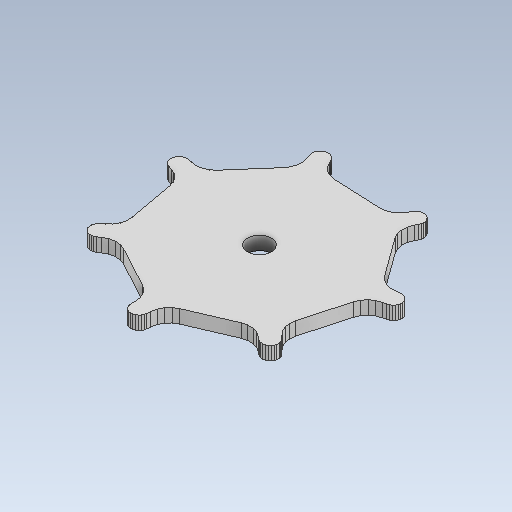
# Autodesk Inventor part: sprocket7
Saved by Autodesk Inventor 2020 (Build 240168000, 168)
## iProperties
Created: 2019-07-16
Part Number: sprocket7
Material: Generic
Document SubType Name: Modeling
Designer: erwin
Density: 1 g/cm^3
Appearance: Default
Mass: 305.43 g
Surface Area: 609.721 cm^2
Volume: 305.43 cm^3
Author: erwin
Autodesk Inventor part; units mm, degrees
ref_plane "YZ Plane" through (0, 0, 0) normal (1, 0, 0) x (0, 1, 0)
ref_plane "XZ Plane" through (0, 0, 0) normal (0, 1, 0) x (-1, 0, 0)
ref_plane "XY Plane" through (0, 0, 0) normal (0, 0, 1) x (1, 0, 0)
sketch "Sketch2" plane through (0, 0, 0) normal (0, 1, 0) x (-1, 0, 0)
  line L0 (77.8598, 129.5505) -> (181.2412, 129.5505)
  line L1 (129.5505, 77.8598) -> (129.5505, 181.2412)
  line L2 (208.1814, 165.1629) -> (207.9893, 170.0518)
  line L3 (207.9893, 170.0518) -> (209.1581, 174.8028)
  line L4 (209.1581, 174.8028) -> (211.5965, 179.0445)
  line L5 (211.5965, 179.0445) -> (215.1139, 182.4454)
  line L6 (215.1139, 182.4454) -> (217.4859, 184.4007)
  line L7 (217.4859, 184.4007) -> (218.8706, 185.7147)
  line L8 (218.8706, 185.7147) -> (219.868, 187.3423)
  line L9 (219.868, 187.3423) -> (220.4102, 189.1727)
  line L10 (220.4102, 189.1727) -> (220.4602, 191.0809)
  line L11 (220.4602, 191.0809) -> (220.0145, 192.9371)
  line L12 (220.0145, 192.9371) -> (219.1037, 194.6147)
  line L13 (219.1037, 194.6147) -> (217.7897, 195.9994)
  line L14 (217.7897, 195.9994) -> (216.162, 196.9968)
  line L15 (216.162, 196.9968) -> (214.3317, 197.5389)
  line L16 (214.3317, 197.5389) -> (212.4235, 197.5889)
  line L17 (212.4235, 197.5889) -> (210.5673, 197.1433)
  line L18 (210.5673, 197.1433) -> (208.8897, 196.2324)
  line L19 (208.8897, 196.2324) -> (206.2971, 194.5807)
  line L20 (206.2971, 194.5807) -> (201.9757, 192.2864)
  line L21 (201.9757, 192.2864) -> (197.1881, 191.2781)
  line L22 (197.1881, 191.2781) -> (192.3084, 191.6346)
  line L23 (192.3084, 191.6346) -> (187.7182, 193.3281)
  line L24 (187.7182, 193.3281) -> (150.7331, 213.2305)
  line L25 (150.7331, 213.2305) -> (146.7911, 216.1285)
  line L26 (146.7911, 216.1285) -> (143.8054, 220.0046)
  line L27 (143.8054, 220.0046) -> (142.0094, 224.5557)
  line L28 (142.0094, 224.5557) -> (141.5435, 229.4261)
  line L29 (141.5435, 229.4261) -> (141.4937, 232.4997)
  line L30 (141.4937, 232.4997) -> (141.3297, 234.4016)
  line L31 (141.3297, 234.4016) -> (140.6791, 236.1962)
  line L32 (140.6791, 236.1962) -> (139.5861, 237.7613)
  line L33 (139.5861, 237.7613) -> (138.1253, 238.9901)
  line L34 (138.1253, 238.9901) -> (136.3963, 239.799)
  line L35 (136.3963, 239.799) -> (134.5168, 240.1329)
  line L36 (134.5168, 240.1329) -> (132.6149, 239.9689)
  line L37 (132.6149, 239.9689) -> (130.8203, 239.3182)
  line L38 (130.8203, 239.3182) -> (129.2552, 238.2252)
  line L39 (129.2552, 238.2252) -> (128.0264, 236.7645)
  line L40 (128.0264, 236.7645) -> (127.2175, 235.0354)
  line L41 (127.2175, 235.0354) -> (126.8836, 233.1559)
  line L42 (126.8836, 233.1559) -> (126.5586, 230.0991)
  line L43 (126.5586, 230.0991) -> (125.658, 225.29)
  line L44 (125.658, 225.29) -> (123.4612, 220.9182)
  line L45 (123.4612, 220.9182) -> (120.1401, 217.3254)
  line L46 (120.1401, 217.3254) -> (115.9541, 214.7925)
  line L47 (115.9541, 214.7925) -> (77.334, 198.2854)
  line L48 (77.334, 198.2854) -> (72.6104, 197.0103)
  line L49 (72.6104, 197.0103) -> (67.7184, 197.0926)
  line L50 (67.7184, 197.0926) -> (63.0404, 198.526)
  line L51 (63.0404, 198.526) -> (58.9421, 201.1984)
  line L52 (58.9421, 201.1984) -> (56.508, 203.0759)
  line L53 (56.508, 203.0759) -> (54.9188, 204.1335)
  line L54 (54.9188, 204.1335) -> (53.1101, 204.7437)
  line L55 (53.1101, 204.7437) -> (51.205, 204.865)
  line L56 (51.205, 204.865) -> (49.3334, 204.4891)
  line L57 (49.3334, 204.4891) -> (47.623, 203.6416)
  line L58 (47.623, 203.6416) -> (46.1901, 202.3802)
  line L59 (46.1901, 202.3802) -> (45.1326, 200.7911)
  line L60 (45.1326, 200.7911) -> (44.5223, 198.9823)
  line L61 (44.5223, 198.9823) -> (44.401, 197.0772)
  line L62 (44.401, 197.0772) -> (44.777, 195.2057)
  line L63 (44.777, 195.2057) -> (45.6245, 193.4952)
  line L64 (45.6245, 193.4952) -> (46.8858, 192.0624)
  line L65 (46.8858, 192.0624) -> (49.073, 189.9023)
  line L66 (49.073, 189.9023) -> (52.2714, 186.1998)
  line L67 (52.2714, 186.1998) -> (54.3197, 181.7566)
  line L68 (54.3197, 181.7566) -> (55.058, 176.9199)
  line L69 (55.058, 176.9199) -> (54.4284, 172.0679)
  line L70 (54.4284, 172.0679) -> (43.2549, 131.5815)
  line L71 (43.2549, 131.5815) -> (41.3067, 127.0934)
  line L72 (41.3067, 127.0934) -> (38.1923, 123.3201)
  line L73 (38.1923, 123.3201) -> (34.1549, 120.5564)
  line L74 (34.1549, 120.5564) -> (29.5103, 119.0184)
  line L75 (29.5103, 119.0184) -> (26.5248, 118.2859)
  line L76 (26.5248, 118.2859) -> (24.7071, 117.7028)
  line L77 (24.7071, 117.7028) -> (23.1023, 116.6692)
  line L78 (23.1023, 116.6692) -> (21.8196, 115.2553)
  line L79 (21.8196, 115.2553) -> (20.9467, 113.5577)
  line L80 (20.9467, 113.5577) -> (20.5428, 111.692)
  line L81 (20.5428, 111.692) -> (20.6356, 109.7853)
  line L82 (20.6356, 109.7853) -> (21.2187, 107.9677)
  line L83 (21.2187, 107.9677) -> (22.2523, 106.3628)
  line L84 (22.2523, 106.3628) -> (23.6661, 105.0802)
  line L85 (23.6661, 105.0802) -> (25.3638, 104.2072)
  line L86 (25.3638, 104.2072) -> (27.2295, 103.8034)
  line L87 (27.2295, 103.8034) -> (29.1361, 103.8961)
  line L88 (29.1361, 103.8961) -> (32.1886, 104.2594)
  line L89 (32.1886, 104.2594) -> (37.0775, 104.4515)
  line L90 (37.0775, 104.4515) -> (41.8285, 103.2827)
  line L91 (41.8285, 103.2827) -> (46.0703, 100.8443)
  line L92 (46.0703, 100.8443) -> (49.4712, 97.3269)
  line L93 (49.4712, 97.3269) -> (74.1582, 63.3482)
  line L94 (74.1582, 63.3482) -> (76.4524, 59.0268)
  line L95 (76.4524, 59.0268) -> (77.4607, 54.2392)
  line L96 (77.4607, 54.2392) -> (77.1042, 49.3595)
  line L97 (77.1042, 49.3595) -> (75.4108, 44.7692)
  line L98 (75.4108, 44.7692) -> (74.122, 41.9784)
  line L99 (74.122, 41.9784) -> (73.4446, 40.1937)
  line L100 (73.4446, 40.1937) -> (73.2521, 38.2945)
  line L101 (73.2521, 38.2945) -> (73.5578, 36.4102)
  line L102 (73.5578, 36.4102) -> (74.3407, 34.6693)
  line L103 (74.3407, 34.6693) -> (75.5476, 33.1902)
  line L104 (75.5476, 33.1902) -> (77.0961, 32.074)
  line L105 (77.0961, 32.074) -> (78.8808, 31.3966)
  line L106 (78.8808, 31.3966) -> (80.78, 31.2041)
  line L107 (80.78, 31.2041) -> (82.6643, 31.5098)
  line L108 (82.6643, 31.5098) -> (84.4053, 32.2927)
  line L109 (84.4053, 32.2927) -> (85.8843, 33.4996)
  line L110 (85.8843, 33.4996) -> (87.0006, 35.0481)
  line L111 (87.0006, 35.0481) -> (88.6197, 37.6612)
  line L112 (88.6197, 37.6612) -> (91.5177, 41.6033)
  line L113 (91.5177, 41.6033) -> (95.3937, 44.589)
  line L114 (95.3937, 44.589) -> (99.9449, 46.385)
  line L115 (99.9449, 46.385) -> (104.8153, 46.8509)
  line L116 (104.8153, 46.8509) -> (146.773, 44.9666)
  line L117 (146.773, 44.9666) -> (151.582, 44.066)
  line L118 (151.582, 44.066) -> (155.9538, 41.8692)
  line L119 (155.9538, 41.8692) -> (159.5466, 38.5481)
  line L120 (159.5466, 38.5481) -> (162.0796, 34.3621)
  line L121 (162.0796, 34.3621) -> (163.458, 31.6144)
  line L122 (163.458, 31.6144) -> (164.431, 29.9721)
  line L123 (164.431, 29.9721) -> (165.7958, 28.6375)
  line L124 (165.7958, 28.6375) -> (167.4596, 27.7016)
  line L125 (167.4596, 27.7016) -> (169.3089, 27.2283)
  line L126 (169.3089, 27.2283) -> (171.2177, 27.2497)
  line L127 (171.2177, 27.2497) -> (173.0559, 27.7644)
  line L128 (173.0559, 27.7644) -> (174.6983, 28.7374)
  line L129 (174.6983, 28.7374) -> (176.0329, 30.1023)
  line L130 (176.0329, 30.1023) -> (176.9687, 31.766)
  line L131 (176.9687, 31.766) -> (177.4421, 33.6153)
  line L132 (177.4421, 33.6153) -> (177.4207, 35.5241)
  line L133 (177.4207, 35.5241) -> (176.9059, 37.3624)
  line L134 (176.9059, 37.3624) -> (175.8725, 40.2575)
  line L135 (175.8725, 40.2575) -> (174.5974, 44.9811)
  line L136 (174.5974, 44.9811) -> (174.6797, 49.873)
  line L137 (174.6797, 49.873) -> (176.1131, 54.551)
  line L138 (176.1131, 54.551) -> (178.7855, 58.6494)
  line L139 (178.7855, 58.6494) -> (206.4189, 90.2784)
  line L140 (206.4189, 90.2784) -> (210.1214, 93.4767)
  line L141 (210.1214, 93.4767) -> (214.5647, 95.5251)
  line L142 (214.5647, 95.5251) -> (219.4013, 96.2633)
  line L143 (219.4013, 96.2633) -> (224.2533, 95.6338)
  line L144 (224.2533, 95.6338) -> (227.261, 94.9983)
  line L145 (227.261, 94.9983) -> (229.1516, 94.735)
  line L146 (229.1516, 94.735) -> (231.046, 94.97)
  line L147 (231.046, 94.97) -> (232.8151, 95.6873)
  line L148 (232.8151, 95.6873) -> (234.3382, 96.838)
  line L149 (234.3382, 96.838) -> (235.5115, 98.3438)
  line L150 (235.5115, 98.3438) -> (236.2552, 100.1018)
  line L151 (236.2552, 100.1018) -> (236.5185, 101.9925)
  line L152 (236.5185, 101.9925) -> (236.2835, 103.8869)
  line L153 (236.2835, 103.8869) -> (235.5662, 105.656)
  line L154 (235.5662, 105.656) -> (234.4155, 107.1791)
  line L155 (234.4155, 107.1791) -> (232.9098, 108.3524)
  line L156 (232.9098, 108.3524) -> (231.1517, 109.0961)
  line L157 (231.1517, 109.0961) -> (228.2439, 110.0932)
  line L158 (228.2439, 110.0932) -> (223.7558, 112.0414)
  line L159 (223.7558, 112.0414) -> (219.9824, 115.1559)
  line L160 (219.9824, 115.1559) -> (217.2187, 119.1932)
  line L161 (217.2187, 119.1932) -> (215.6807, 123.8378)
  line L162 (215.6807, 123.8378) -> (208.1814, 165.1629)
  circle A0 centre (129.5505, 129.5505) radius 10.75
  dimension "d0" = 21.5
  constraints: 326 end point, 1 centre point, 1 midpoint
  measures "d0" diameter of A0
extrude "Extrusion1" add sketch "Sketch2" along normal blind 12
body "Solid1"
